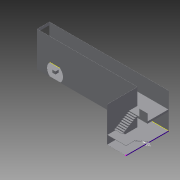
# Autodesk Inventor part: ATF_Corridors_Drawing
Saved by Autodesk Inventor 2013 SP2 (Build 170200200, 200)
## iProperties
Created: 2014-01-16
Part Number: ATF_Corridors_Drawing
Material: Generic
Document SubType Name: Modeling
Designer: mcgratta
Density: 1 g/cm^3
Author: mcgratta
Autodesk Inventor part; units mm, degrees
ref_plane "YZ Plane" through (0, 0, 0) normal (1, 0, 0) x (0, 1, 0)
ref_plane "XZ Plane" through (0, 0, 0) normal (0, 1, 0) x (-1, 0, 0)
ref_plane "XY Plane" through (0, 0, 0) normal (0, 0, 1) x (1, 0, 0)
sketch "Sketch1" plane through (0, 0, 0) normal (0, 1, 0) x (-1, 0, 0)
  line L0 (0, 0) -> (14380, 0)
  line L1 (14380, 0) -> (14380, -1790)
  line L2 (14380, -1790) -> (0, -1790)
  line L3 (0, -1790) -> (0, 0)
  line L4 (0, -1790) -> (-2720, -1790)
  line L5 (-2720, -1790) -> (-2720, 4350)
  line L6 (-2720, 4350) -> (0, 4350)
  line L7 (0, 4350) -> (0, -1790)
  dimension "d0" = 1790
  dimension "d2" = 14380
  dimension "d3" = 2720
  dimension "d4" = 6140
  constraints: 16 end point, 4 parallel, 2 horizontal, 2 perpendicular
  measures "d0" distance between parallel lines of L0 L2
  measures "d2" distance between parallel lines of L3 L1
  measures "d3" distance between parallel lines of L5 L7
  measures "d4" distance between parallel lines of L6 L4
extrude "Extrusion1" add sketch "Sketch1" along normal blind 10
sketch "Sketch2" plane through (0, 10, 0) normal (0, 1, 0) x (1, 0, 0)
  line L0 (2720, -4350) -> (2720, 1790) projected
  line L1 (0, -4350) -> (2720, -4350)
  line L2 (2720, -4350) -> (2720, -4330)
  line L3 (2720, -4330) -> (0, -4330)
  line L4 (0, -4330) -> (0, -4350)
  dimension "d7" = 20
  constraints: 8 end point, 2 parallel, 1 horizontal, 1 perpendicular, 1 point on line
  measures "d7" distance between parallel lines of L3 L1
extrude "Extrusion2" [suppressed]
sketch "Sketch3" plane through (0, 10, 0) normal (0, 1, 0) x (1, 0, 0)
  line L0 (2720, 1790) -> (-14380, 1790) projected
  line L1 (2720, -4330) -> (2700, -4330)
  line L2 (2700, -4330) -> (2700, 1790)
  line L3 (2700, 1790) -> (2720, 1790)
  line L4 (2720, 1790) -> (2720, -4330)
  dimension "d11" = 20
  constraints: 8 end point, 2 parallel, 1 horizontal, 1 perpendicular, 1 point on line
  measures "d11" distance between parallel lines of L4 L2
sketch "Sketch4" plane through (0, 10, 0) normal (0, 1, 0) x (1, 0, 0)
  line L0 (-14380, 1790) -> (-14380, 0) projected
  line L1 (2700, 1790) -> (-14380, 1790)
  line L2 (-14380, 1790) -> (-14380, 1770)
  line L3 (-14380, 1770) -> (2700, 1770)
  line L4 (2700, 1770) -> (2700, 1790)
  dimension "d15" = 20
  constraints: 8 end point, 2 parallel, 1 horizontal, 1 perpendicular, 1 point on line
  measures "d15" distance between parallel lines of L3 L1
extrude "Extrusion4" add sketch "Sketch4" along normal blind 5000
sketch "Sketch5" plane through (0, 10, 0) normal (0, 1, 0) x (1, 0, 0)
  line L0 (-14380, 0) -> (0, 0) projected
  line L1 (-14380, 1770) -> (-14360, 1770)
  line L2 (-14360, 1770) -> (-14360, 0)
  line L3 (-14360, 0) -> (-14380, 0)
  line L4 (-14380, 0) -> (-14380, 1770)
  dimension "d19" = 20
  constraints: 8 end point, 2 parallel, 1 horizontal, 1 perpendicular, 1 point on line
  measures "d19" distance between parallel lines of L2 L4
extrude "Extrusion5" add sketch "Sketch5" along normal blind 5000
sketch "Sketch6" plane through (0, 10, 0) normal (0, 1, 0) x (1, 0, 0)
  line L0 (-14360, 0) -> (0, 0)
  line L1 (0, 0) -> (0, 20)
  line L2 (0, 20) -> (-14360, 20)
  line L3 (-14360, 20) -> (-14360, 0)
  dimension "d23" = 20
  constraints: 8 end point, 2 parallel, 1 horizontal, 1 perpendicular
  measures "d23" distance between parallel lines of L0 L2
extrude "Extrusion6" add sketch "Sketch6" along normal blind 5000
sketch "Sketch7" plane through (0, 10, 0) normal (0, 1, 0) x (1, 0, 0)
  line L0 (0, 0) -> (0, -4350) projected
  line L1 (0, -4330) -> (2720, -4330) projected
  line L2 (0, 0) -> (20, 0)
  line L3 (20, 0) -> (20, -4330)
  line L4 (20, -4330) -> (0, -4330)
  line L5 (0, -4330) -> (0, 0)
  point P0 (2700, -4330)
  dimension "d27" = 20
  constraints: 8 end point, 2 parallel, 1 horizontal, 1 perpendicular, 1 point on line
  measures "d27" distance between parallel lines of L3 L5
extrude "Extrusion7" add sketch "Sketch7" along normal blind 5000
ref_plane "Work Plane1" through (2690, 10, 4330) normal (-1, 0, 0) x (0, 0, 1)
sketch "Sketch10" plane through (2690, 10, 4330) normal (-1, 0, 0) x (0, 0, 1)
  line L0 (-3212, 172.1) -> (-2978, 172.1)
  line L1 (-2978, 172.1) -> (-2978, 134)
  line L2 (-2978, 134) -> (-3212, 134)
  line L3 (-3212, 134) -> (-3212, 172.1)
  line L4 (-6120, -10) -> (-6120, 5000) projected
  line L5 (-4330, 0) -> (20, 0) projected
  line L6 (-2978, 306.1) -> (-2744, 306.1)
  line L7 (-2744, 306.1) -> (-2744, 268)
  line L8 (-2744, 268) -> (-2978, 268)
  line L9 (-2978, 268) -> (-2978, 306.1)
  line L10 (-2744, 440.1) -> (-2510, 440.1)
  line L11 (-2510, 440.1) -> (-2510, 402)
  line L12 (-2510, 402) -> (-2744, 402)
  line L13 (-2744, 402) -> (-2744, 440.1)
  line L14 (-2510, 574.1) -> (-2276, 574.1)
  line L15 (-2276, 574.1) -> (-2276, 536)
  line L16 (-2276, 536) -> (-2510, 536)
  line L17 (-2510, 536) -> (-2510, 574.1)
  line L18 (-2276, 708.1) -> (-2042, 708.1)
  line L19 (-2042, 708.1) -> (-2042, 670)
  line L20 (-2042, 670) -> (-2276, 670)
  line L21 (-2276, 670) -> (-2276, 708.1)
  line L22 (-2042, 842.1) -> (-1808, 842.1)
  line L23 (-1808, 842.1) -> (-1808, 804)
  line L24 (-1808, 804) -> (-2042, 804)
  line L25 (-2042, 804) -> (-2042, 842.1)
  line L26 (-1808, 976.1) -> (-1574, 976.1)
  line L27 (-1574, 976.1) -> (-1574, 938)
  line L28 (-1574, 938) -> (-1808, 938)
  line L29 (-1808, 938) -> (-1808, 976.1)
  line L30 (-1574, 1110.1) -> (-1340, 1110.1)
  line L31 (-1340, 1110.1) -> (-1340, 1072)
  line L32 (-1340, 1072) -> (-1574, 1072)
  line L33 (-1574, 1072) -> (-1574, 1110.1)
  point P0 (-4330, -10)
  point P1 (0, 0)
  dimension "d74" = 38.1
  dimension "d76" = 2908
  dimension "d77" = 234
  dimension "d78" = 134
  dimension "d79" = 38.1
  dimension "d80" = 234
  dimension "d81" = 0
  dimension "d82" = 134
  dimension "d83" = 38.1
  dimension "d84" = 234
  dimension "d85" = 38.1
  dimension "d86" = 234
  dimension "d87" = 0
  dimension "d88" = 134
  dimension "d89" = 0
  dimension "d90" = 134
  dimension "d91" = 38.1
  dimension "d92" = 234
  dimension "d93" = 38.1
  dimension "d94" = 234
  dimension "d95" = 0
  dimension "d96" = 134
  dimension "d97" = 38.1
  dimension "d98" = 234
  dimension "d99" = 38.1
  dimension "d100" = 234
  dimension "d101" = 0
  dimension "d102" = 134
  dimension "d103" = 0
  dimension "d104" = 134
  dimension "d105" = 0
  dimension "d106" = 134
  constraints: 64 end point, 16 parallel, 8 horizontal, 8 perpendicular
  measures "d74" distance between parallel lines of L2 L0
  measures "d76" distance from line of L4 L0.start
  measures "d77" distance of L0.end L0.start
  measures "d78" distance between parallel lines of L5 L2
  measures "d79" distance between parallel lines of L8 L6
  measures "d80" distance of L6.end L6.start
  measures "d81" distance between parallel lines of L9 L1
  measures "d82" distance between parallel lines of L2 L8
  measures "d83" distance between parallel lines of L12 L10
  measures "d84" distance of L10.end L10.start
  measures "d85" distance between parallel lines of L16 L14
  measures "d86" distance of L14.end L14.start
  measures "d87" distance between parallel lines of L17 L11
  measures "d88" distance between parallel lines of L12 L16
  measures "d89" distance from line of L7.end L13
  measures "d90" distance between parallel lines of L8 L12
  measures "d91" distance between parallel lines of L20 L18
  measures "d92" distance of L19.start L21.end
  measures "d93" distance between parallel lines of L24 L22
  measures "d94" distance of L23.start L25.end
  measures "d95" distance between parallel lines of L25 L19
  measures "d96" distance between parallel lines of L20 L24
  measures "d97" distance between parallel lines of L28 L26
  measures "d98" distance of L26.end L29.end
  measures "d99" distance between parallel lines of L32 L30
  measures "d100" distance of L30.end L33.end
  measures "d101" distance between parallel lines of L33 L27
  measures "d102" distance between parallel lines of L28 L32
  measures "d103" distance from line of L23.end L29
  measures "d104" distance between parallel lines of L24 L28
  measures "d105" distance between parallel lines of L21 L15
  measures "d106" distance between parallel lines of L16 L20
extrude "Extrusion10" add sketch "Sketch10" along normal blind 1136
sketch "Sketch11" plane through (2690, 10, 4330) normal (-1, 0, 0) x (0, 0, 1)
  line L0 (-1340, 1210) -> (-10, 1210)
  line L1 (-10, 1210) -> (-10, 1171.9)
  line L2 (-10, 1171.9) -> (-1340, 1171.9)
  line L3 (-1340, 1171.9) -> (-1340, 1210)
  line L4 (-1340, 1072) -> (-1340, 1110.1) projected
  line L5 (0, 0) -> (0, 5000) projected
  line L6 (-4330, 0) -> (20, 0) projected
  point P0 (-4330, -10)
  dimension "d109" = 0
  dimension "d110" = 10
  dimension "d111" = 38.1
  dimension "d112" = 1210
  constraints: 8 end point, 2 parallel, 1 horizontal, 1 perpendicular
  measures "d109" distance from line of L0.start L4
  measures "d110" distance from line of L5 L0.end
  measures "d111" distance between parallel lines of L2 L0
  measures "d112" distance between parallel lines of L6 L0
extrude "Extrusion11" add sketch "Sketch11" along normal blind 2660
sketch "Sketch12" plane through (0, 10, 0) normal (0, 1, 0) x (1, 0, 0)
  line L0 (-14360, 1770) -> (-14360, 20) projected
  line L1 (-14360, 20) -> (0, 20) projected
  line L2 (-12860, 1120) -> (-12410, 1120)
  line L3 (-12410, 1120) -> (-12410, 670)
  line L4 (-12410, 670) -> (-12860, 670)
  line L5 (-12860, 670) -> (-12860, 1120)
  dimension "d115" = 1500
  dimension "d116" = 450
  dimension "d117" = 450
  dimension "d118" = 650
  constraints: 8 end point, 2 parallel, 1 horizontal, 1 perpendicular
  measures "d115" distance between parallel lines of L5 L0
  measures "d116" distance between parallel lines of L4 L2
  measures "d117" distance between parallel lines of L3 L5
  measures "d118" distance between parallel lines of L1 L4
extrude "Extrusion12" add sketch "Sketch12" along normal blind 370
sketch "Sketch13" plane through (-14360, 10, -1770) normal (1, 0, 0) x (0, 0, -1)
  line L0 (-1750, 5000) -> (-1750, 0) projected
  line L1 (0, 0) -> (-1750, 0) projected
  line L2 (0, 5000) -> (0, 0) projected
  line L3 (-1750, 5000) -> (0, 5000) projected
  line L4 (-1750, 2650) -> (0, 2650)
  line L5 (0, 2650) -> (0, 2370)
  line L6 (0, 2370) -> (-1750, 2370)
  line L7 (-1750, 2370) -> (-1750, 2650)
  point P0 (-1770, -10)
  dimension "d121" = 2370
  dimension "d122" = 2350
  constraints: 8 end point, 2 parallel, 2 point on line, 1 horizontal, 1 perpendicular
  measures "d121" distance between parallel lines of L1 L6
  measures "d122" distance between parallel lines of L4 L3
extrude "Extrusion13" add sketch "Sketch13" along normal blind 17040 contours L4 L2 L6 L0
sketch "Sketch14" plane through (0, 2380, -20) normal (0, 0, 1) x (1, 0, 0)
  line L0 (0, 0) -> (0, 280) projected
  line L1 (0, 0) -> (2680, 0) projected
  line L2 (0, 280) -> (2680, 280)
  line L3 (2680, 280) -> (2680, 0)
  line L4 (2680, 0) -> (0, 0)
  line L5 (0, 0) -> (0, 280)
  point P0 (0, -2380)
  constraints: 8 end point, 2 parallel, 1 horizontal, 1 perpendicular
extrude "Extrusion14" add sketch "Sketch14" along normal blind 1239
sketch "Sketch15" plane through (20, 10, 4330) normal (1, 0, 0) x (0, 0, -1)
  line L0 (3111, 2650) -> (4330, 2650) projected
  line L1 (3111, 2370) -> (3111, 2650) projected
  line L2 (2877, 2516) -> (3111, 2516)
  line L3 (3111, 2516) -> (3111, 2477.9)
  line L4 (3111, 2477.9) -> (2877, 2477.9)
  line L5 (2877, 2477.9) -> (2877, 2516)
  line L6 (2643, 2382) -> (2877, 2382)
  line L7 (2877, 2382) -> (2877, 2343.9)
  line L8 (2877, 2343.9) -> (2643, 2343.9)
  line L9 (2643, 2343.9) -> (2643, 2382)
  line L10 (2409, 2248) -> (2643, 2248)
  line L11 (2643, 2248) -> (2643, 2209.9)
  line L12 (2643, 2209.9) -> (2409, 2209.9)
  line L13 (2409, 2209.9) -> (2409, 2248)
  line L14 (2175, 2114) -> (2409, 2114)
  line L15 (2409, 2114) -> (2409, 2075.9)
  line L16 (2409, 2075.9) -> (2175, 2075.9)
  line L17 (2175, 2075.9) -> (2175, 2114)
  line L18 (1941, 1980) -> (2175, 1980)
  line L19 (2175, 1980) -> (2175, 1941.9)
  line L20 (2175, 1941.9) -> (1941, 1941.9)
  line L21 (1941, 1941.9) -> (1941, 1980)
  line L22 (1941, 1820.2689) -> (1941, 1782.1689)
  line L23 (1707, 1782.1689) -> (1707, 1820.2689)
  line L24 (1707, 1820.2689) -> (1941, 1820.2689)
  line L25 (1941, 1782.1689) -> (1707, 1782.1689)
  line L26 (1707, 1686.2689) -> (1707, 1648.1689)
  line L27 (1473, 1648.1689) -> (1473, 1686.2689)
  line L28 (1473, 1686.2689) -> (1707, 1686.2689)
  line L29 (1707, 1648.1689) -> (1473, 1648.1689)
  line L30 (1473, 1552.2689) -> (1473, 1514.1689)
  line L31 (1239, 1514.1689) -> (1239, 1552.2689)
  line L32 (1239, 1552.2689) -> (1473, 1552.2689)
  line L33 (1473, 1514.1689) -> (1239, 1514.1689)
  line L34 (1239, 1418.2689) -> (1239, 1380.1689)
  line L35 (1005, 1418.2689) -> (1239, 1418.2689)
  line L36 (1239, 1380.1689) -> (1005, 1380.1689)
  line L37 (1005, 1380.1689) -> (1005, 1418.2689)
  point P0 (4330, -10)
  dimension "d127" = 234
  dimension "d129" = 0
  dimension "d130" = 134
  dimension "d131" = 38.1
  dimension "d132" = 234
  dimension "d133" = 38.1
  dimension "d134" = 0
  dimension "d135" = 134
  dimension "d136" = 234
  dimension "d137" = 38.1
  dimension "d138" = 234
  dimension "d139" = 38.1
  dimension "d140" = 234
  dimension "d141" = 38.1
  dimension "d142" = 0
  dimension "d143" = 0
  dimension "d144" = 0
  dimension "d145" = 134
  dimension "d146" = 134
  dimension "d147" = 134
  dimension "d148" = 234
  dimension "d149" = 38.1
  dimension "d150" = 234
  dimension "d151" = 38.1
  dimension "d152" = 234
  dimension "d153" = 38.1
  dimension "d154" = 0
  dimension "d155" = 0
  dimension "d156" = 134
  dimension "d157" = 134
  dimension "d158" = 0
  dimension "d159" = 159.7311
  dimension "d162" = 234
  dimension "d163" = 38.1
  dimension "d164" = 0
  dimension "d165" = 134
  constraints: 72 end point, 18 parallel, 9 horizontal, 9 perpendicular
  measures "d127" distance between parallel lines of L3 L5
  measures "d129" distance between parallel lines of L3 L1
  measures "d130" distance between parallel lines of L2 L0
  measures "d131" distance between parallel lines of L4 L2
  measures "d132" distance between parallel lines of L7 L9
  measures "d133" distance between parallel lines of L8 L6
  measures "d134" horizontal distance of L4.end L7.end
  measures "d135" distance between parallel lines of L4 L8
  measures "d136" distance between parallel lines of L11 L13
  measures "d137" distance between parallel lines of L12 L10
  measures "d138" distance between parallel lines of L15 L17
  measures "d139" distance between parallel lines of L16 L14
  measures "d140" distance between parallel lines of L19 L21
  measures "d141" distance between parallel lines of L20 L18
  measures "d142" horizontal distance of L6.start L11.end
  measures "d143" horizontal distance of L13.end L15.end
  measures "d144" horizontal distance of L17.end L19.start
  measures "d145" distance between parallel lines of L12 L8
  measures "d146" distance between parallel lines of L12 L16
  measures "d147" distance between parallel lines of L16 L20
  measures "d148" distance between parallel lines of L22 L23
  measures "d149" distance between parallel lines of L25 L24
  measures "d150" distance between parallel lines of L26 L27
  measures "d151" distance between parallel lines of L29 L28
  measures "d152" distance between parallel lines of L30 L31
  measures "d153" distance between parallel lines of L33 L32
  measures "d154" horizontal distance of L24.start L26.end
  measures "d155" horizontal distance of L28.start L30.start
  measures "d156" distance between parallel lines of L25 L29
  measures "d157" distance between parallel lines of L29 L33
  measures "d158" horizontal distance of L21.start L25.start
  measures "d159" distance between parallel lines of L20 L25
  measures "d162" distance between parallel lines of L34 L37
  measures "d163" distance between parallel lines of L36 L35
  measures "d164" distance between parallel lines of L34 L31
  measures "d165" distance between parallel lines of L36 L33
extrude "Extrusion16" add sketch "Sketch15" along normal blind 1150
sketch "Sketch16" plane through (-14360, 2660, -20) normal (0, 1, 0) x (1, 0, 0)
  line L0 (17040, -1239) -> (15884, -1239)
  line L1 (15884, -1239) -> (15884, -1219)
  line L2 (15884, -1219) -> (17040, -1219)
  line L3 (17040, -1219) -> (17040, -1239)
  dimension "d168" = 20
  dimension "d170" = 1156
  constraints: 8 end point, 2 parallel, 1 horizontal, 1 perpendicular
  measures "d168" distance between parallel lines of L2 L0
  measures "d170" distance of L2.end L1.end
extrude "Extrusion17" add sketch "Sketch16" along normal blind 1000
sketch "Sketch17" plane through (-14380, 0, -1790) normal (-1, 0, 0) x (0, 0, 1)
  line L0 (0, 5010) -> (1790, 5010) projected
  line L1 (20, 2663) -> (1770, 2663)
  line L2 (1770, 2663) -> (1770, 4619)
  line L3 (1770, 4619) -> (20, 4619)
  line L4 (20, 4619) -> (20, 2663)
  line L5 (0, 0) -> (0, 5010) projected
  dimension "d179" = 20
  dimension "d180" = 1750
  dimension "d181" = 391
  dimension "d182" = 1956
  constraints: 8 end point, 2 parallel, 1 horizontal, 1 perpendicular
  measures "d179" distance between parallel lines of L5 L4
  measures "d180" distance between parallel lines of L2 L4
  measures "d181" distance between parallel lines of L3 L0
  measures "d182" distance between parallel lines of L1 L3
extrude "Extrusion18" cut sketch "Sketch17" along normal mid plane 50
sketch "Sketch18" plane through (-14380, 0, 0) normal (0, 0, 1) x (1, 0, 0)
  line L0 (0, 0) -> (14380, 0) projected
  arc A0 (3305.7392, 0) -> (1827.2099, 0) centre (2566.4746, 886.2602) ccw
  constraints: 2 point on circle, 2 point on line, 1 centre point
extrude "Extrusion19" cut sketch "Sketch18" along normal mid plane 50
body "Solid1"
